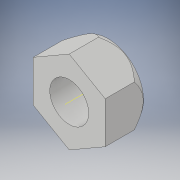
# Autodesk Inventor part: nut M12
Saved by Autodesk Inventor 2018 (Build 220112000, 112)
## iProperties
Created: 2021-03-15
Part Number: nut M12
Material: Generic
Document SubType Name: Modeling
Designer: Jyoti Soni
Density: 1 g/cm^3
Appearance: Default
Author: Jyoti Soni
Autodesk Inventor part; units mm, degrees
ref_plane "YZ Plane" through (0, 0, 0) normal (1, 0, 0) x (0, 1, 0)
ref_plane "XZ Plane" through (0, 0, 0) normal (0, 1, 0) x (-1, 0, 0)
ref_plane "XY Plane" through (0, 0, 0) normal (0, 0, 1) x (1, 0, 0)
sketch "Sketch2" plane through (0, 0, 0) normal (0, 0, 1) x (1, 0, 0)
  line L0 (0, 12.7947) -> (11.0805, 6.3973)
  line L1 (11.0805, 6.3973) -> (11.0805, -6.3973)
  line L2 (11.0805, -6.3973) -> (0, -12.7947)
  line L3 (0, -12.7947) -> (-11.0805, -6.3973)
  line L4 (-11.0805, -6.3973) -> (-11.0805, 6.3973)
  line L5 (-11.0805, 6.3973) -> (0, 12.7947)
  circle A0 centre (0, 0) radius 6
  dimension "d0" = 12
  constraints: 12 end point, 2 coincident, 1 centre point, 13 other
  measures "d0" diameter of A0
extrude "Extrusion1" add sketch "Sketch2" along normal blind 12
sketch "Sketch5" plane through (0, 0, 0) normal (1, 0, 0) x (0, 1, 0)
  line L0 (13.8205, 4.649) -> (13.8205, -1.691)
  line L1 (13.8205, -1.691) -> (9.8308, -1.691)
  line L2 (9.8308, -1.691) -> (13.8205, 4.649)
  line L3 (0, -4.894) -> (0, 14.8157) projected
  point P0 (0, 0)
  constraints: 6 end point, 1 perpendicular, 1 vertical
revolve "Revolution1" cut sketch "Sketch5" angle 360 about axis through (0, 0, 0) along (0, 0, 1)
body "Solid1"
